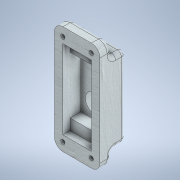
# Autodesk Inventor part: ramie03-5
Saved by Autodesk Inventor 2021 (Build 250183000, 183)
## iProperties
Created: 2021-11-08
Part Number: ramie03-5
Material: Generic
Document SubType Name: Modeling
Designer: Łukasz
Density: 1 g/cm^3
Appearance: Wood - Painted White
Author: Łukasz
Autodesk Inventor part; units mm, degrees
ref_plane "YZ Plane" through (0, 0, 0) normal (1, 0, 0) x (0, 1, 0)
ref_plane "XZ Plane" through (0, 0, 0) normal (0, 1, 0) x (-1, 0, 0)
ref_plane "XY Plane" through (0, 0, 0) normal (0, 0, 1) x (1, 0, 0)
sketch "Sketch1" plane through (0, 0, 0) normal (0, 0, 1) x (1, 0, 0)
  line L0 (0, 0) -> (-32, 0)
  line L1 (-32, 0) -> (-32, 76)
  line L2 (-32, 76) -> (0, 76)
  line L3 (0, 76) -> (0, 0)
  dimension "d0" = 32
  dimension "d1" = 76
  constraints: 8 end point, 2 parallel, 1 horizontal, 1 perpendicular
  measures "d0" distance of L1.end L2.end
  measures "d1" distance of L0.end L1.end
extrude "Extrusion1" add sketch "Sketch1" along normal blind 18
fillet "Fillet1" radius 6 4 edges at (0, 76, 9) (-32, 76, 9) (0, 0, 9) (-32, 0, 9)
sketch "Sketch2" plane through (0, 0, 18) normal (0, 0, 1) x (1, 0, 0)
  line L0 (-6, 58) -> (-26, 58)
  line L1 (-26, 58) -> (-26, 18)
  line L2 (-26, 18) -> (-6, 18)
  line L3 (-6, 18) -> (-6, 58)
  line L4 (-6, 76) -> (-26, 76) projected
  line L5 (0, 6) -> (0, 70) projected
  point P0 (0, 0)
  dimension "d5" = 20
  dimension "d6" = 40
  dimension "d7" = 18
  dimension "d8" = 6
  constraints: 8 end point, 2 parallel, 1 horizontal, 1 perpendicular
  measures "d5" distance of L2.end L1.end
  measures "d6" distance of L1.end L0.end
  measures "d7" distance between parallel lines of L4 L0
  measures "d8" distance between parallel lines of L5 L3
extrude "Extrusion2" cut sketch "Sketch2" against normal blind 12.5
sketch "Sketch3" plane through (0, 0, 5.5) normal (0, 0, 1) x (1, 0, 0)
  circle A0 centre (-16, 28) radius 6.75
  line L0 (-6, 58) -> (-6, 18) projected
  line L1 (-6, 18) -> (-26, 18) projected
  point P0 (0, 0)
  dimension "d11" = 13.5
  dimension "d12" = 10
  dimension "d13" = 10
  constraints: 1 centre point
  measures "d11" diameter of A0
  measures "d12" distance from line of L0 A0.centre
  measures "d13" distance from line of L1 A0.centre
extrude "Extrusion3" cut sketch "Sketch3" against normal up to surface (5.5 mm away)
sketch "Sketch4" plane through (0, 0, 18) normal (0, 0, 1) x (1, 0, 0)
  line L0 (-26, 58) -> (-6, 58) projected
  line L1 (-6, 58) -> (-26, 58)
  line L2 (-26, 58) -> (-26, 65.7)
  line L3 (-26, 65.7) -> (-6, 65.7)
  line L4 (-6, 65.7) -> (-6, 58)
  line L5 (-6, 18) -> (-26, 18) projected
  line L6 (-6, 18) -> (-26, 18)
  line L7 (-26, 18) -> (-26, 10.3)
  line L8 (-26, 10.3) -> (-6, 10.3)
  line L9 (-6, 10.3) -> (-6, 18)
  point P0 (0, 0)
  point P1 (-26, 18)
  dimension "d16" = 7.7
  dimension "d17" = 20
  dimension "d18" = 7.7
  constraints: 16 end point, 4 parallel, 2 horizontal, 2 perpendicular
  measures "d16" distance of L1.end L2.end
  measures "d17" distance of L8.end L7.end
  measures "d18" distance of L7.end L6.end
extrude "Extrusion4" cut sketch "Sketch4" against normal blind 5
sketch "Sketch5" plane through (0, 6, 0) normal (1, 0, 0) x (0, 0, -1)
  line L0 (0, -6) -> (-18, -6) projected
  line L1 (0, -6) -> (0, 4)
  line L2 (0, 0) -> (0, -6) projected
  line L3 (0, 4) -> (-10, 4)
  line L4 (-10, 4) -> (-10, -6)
  line L5 (0, 70) -> (0, 64) projected
  line L6 (0, 70) -> (-10, 70)
  line L7 (-10, 70) -> (-10, 60)
  line L8 (-10, 60) -> (0, 60)
  line L9 (0, 60) -> (0, 70)
  dimension "d21" = 10
  dimension "d22" = 10
  dimension "d23" = 10
  dimension "d24" = 10
  constraints: 14 end point, 3 perpendicular, 2 parallel, 1 collinear, 1 horizontal
  measures "d21" distance of L0.start L1.end
  measures "d22" distance of L1.end L3.end
  measures "d23" distance of L8.end L7.end
  measures "d24" distance of L7.end L6.end
extrude "Extrusion5" cut sketch "Sketch5" against normal up to surface (32 mm away)
fillet "Fillet2" radius 3 20 edges at (-16, 66, 0) (0, 38, 0) (-16, 10, 0) (-32, 38, 0) (0, 66, 5) (-32, 66, 5) (0, 10, 5) (-16, 66, 10) (-32, 10, 5) (-16, 10, 10) (-16, 76, 10) (-30.2426, 74.2426, 10) (-32, 68, 10) (0, 68, 10) (-1.7574, 74.2426, 10) (-1.7574, 1.7574, 10) (0, 8, 10) (-30.2426, 1.7574, 10) (-32, 8, 10) (-16, 0, 10)
sketch "Sketch6" plane through (-3, 69, 10) normal (0, 0, -1) x (-1, 0, 0)
  arc A0 (26, 1) -> (23, 4) centre (23, 1) ccw projected
  circle A1 centre (23, 1) radius 1.5
  arc A2 (3, 4) -> (0, 1) centre (3, 1) ccw projected
  circle A3 centre (3, 1) radius 1.5
  arc A4 (0, -63) -> (3, -66) centre (3, -63) ccw projected
  circle A5 centre (3, -63) radius 1.5
  arc A6 (23, -66) -> (26, -63) centre (23, -63) ccw projected
  circle A7 centre (23, -63) radius 1.5
  point P0 (-3, -69)
  dimension "d28" = 3
  dimension "d29" = 3
  dimension "d30" = 3
  dimension "d31" = 3
  constraints: 4 centre point, 4 coincident
  measures "d28" diameter of A1
  measures "d29" diameter of A3
  measures "d30" diameter of A5
  measures "d31" diameter of A7
extrude "Extrusion6" cut sketch "Sketch6" along normal blind 5 and the other way blind 10
body "Solid1"
